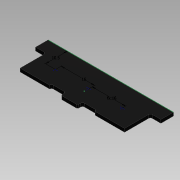
# Autodesk Inventor part: AK-C-C39-Insert-Board
Saved by Autodesk Inventor 2016 (Build 200138000, 138)
## iProperties
Created: 2016-04-01
Part Number: AK-C-C39-Insert-Board
Material: Generic
Document SubType Name: Modeling
Designer: admin
Density: 1 g/cm^3
Appearance: Glossy - Black
Author: admin
Autodesk Inventor part; units mm, degrees
ref_plane "YZ Plane" through (0, 0, 0) normal (1, 0, 0) x (0, 1, 0)
ref_plane "XZ Plane" through (0, 0, 0) normal (0, 1, 0) x (-1, 0, 0)
ref_plane "XY Plane" through (0, 0, 0) normal (0, 0, 1) x (1, 0, 0)
sketch "Sketch1" plane through (0, 0, 0) normal (0, 0, 1) x (1, 0, 0)
  line L0 (-30, 12.6375) -> (30, 12.6375)
  line L1 (30, 12.6375) -> (30, 6.6375)
  line L2 (30, 6.6375) -> (25.875, 6.6375)
  line L3 (25, 5.7625) -> (25, -5.7625)
  line L4 (25, -5.7625) -> (10.875, -5.7625)
  line L5 (4, -5.7625) -> (4, -6.7625)
  line L6 (3.5, -7.2625) -> (-3.5, -7.2625)
  line L7 (-4, -6.7625) -> (-4, -5.7625)
  line L8 (-10.875, -5.7625) -> (-25, -5.7625)
  line L9 (-25, -5.7625) -> (-25, 5.7625)
  line L10 (-25.875, 6.6375) -> (-30, 6.6375)
  line L11 (-30, 6.6375) -> (-30, 12.6375)
  arc A0 (-4, -5.7625) -> (-4.875, -4.8875) centre (-4.875, -5.7625) ccw
  arc A1 (4.875, -4.8875) -> (4, -5.7625) centre (4.875, -5.7625) ccw
  arc A2 (-25, 5.7625) -> (-25.875, 6.6375) centre (-25.875, 5.7625) ccw
  arc A3 (25.875, 6.6375) -> (25, 5.7625) centre (25.875, 5.7625) ccw
  line L12 (0, 4.2796) -> (0, -4.2796) construction
  line L13 (-9.9053, 0) -> (11.8635, 0) construction
  line L14 (-4, -6.7625) -> (-3.5, -7.2625)
  line L15 (3.5, -7.2625) -> (4, -6.7625)
  arc A4 (-10, -4.8875) -> (-10.875, -5.7625) centre (-10, -5.7625) ccw
  arc A5 (10.875, -5.7625) -> (10, -4.8875) centre (10, -5.7625) ccw
  line L16 (-10, -4.8875) -> (-4.875, -4.8875)
  line L17 (4.875, -4.8875) -> (10, -4.8875)
  point P0 (0, 0)
  point P1 (0, 12.6375)
  point P2 (-25, 0)
  dimension "d0" = 1.75
  dimension "d3" = 1.5
  dimension "d5" = 6
  dimension "d6" = 5
  dimension "d11" = 25
  dimension "d12" = 45
  dimension "d13" = 0.5
  dimension "d14" = 8
  dimension "d16" = 18.4
  dimension "d17" = 6
  constraints: 36 end point, 13 point on circle, 11 perpendicular, 8 tangent, 7 point on line, 6 centre point, 5 equal radius, 5 horizontal, 3 midpoint, 2 equal length, 1 collinear, 1 horizontal alignment, 1 vertical, 1 vertical alignment, 2 other
  measures "d0" diameter of A0
  measures "d3" distance between parallel lines of L6 L8
  measures "d5" distance between parallel lines of L2 L0
  measures "d6" distance between parallel lines of L9 L11
  measures "d11" distance between parallel lines of L9 L12
  measures "d12" angle of L6 L14
  measures "d13" distance from line of L6.end L7
  measures "d14" distance between parallel lines of L5 L7
  measures "d16" distance between parallel lines of L0 L4
  measures "d17" distance from line of A4.centre L7
extrude "Extrusion1" add sketch "Sketch1" along normal blind 1.6
sketch "Sketch2" plane through (0, 0, 1.6) normal (0, 0, 1) x (1, 0, 0)
  line L0 (30, 12.6375) -> (-30, 12.6375) projected
  point P0 (0, 0)
  point P1 (-16, 2.1375)
  point P2 (0, 2.1375)
  point P3 (16, 2.1375)
  dimension "d9" = 16
  dimension "d10" = 16
  dimension "d15" = 10.5
  constraints: 2 horizontal alignment, 1 vertical alignment
  measures "d9" distance of point (0, 2.137) point (-16, 2.137)
  measures "d10" distance of point (16, 2.137) point (0, 2.137)
  measures "d15" distance from line of L0 point (-16, 2.137)
equation "\"d10\" = d9"
body "Solid1"
